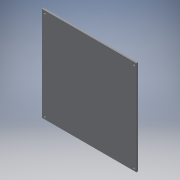
# Autodesk Inventor part: heated-bed
Saved by Autodesk Inventor 2018 (Build 220112000, 112)
## iProperties
Created: 2017-10-01
Part Number: heated-bed
Material: Generic
Document SubType Name: Modeling
Designer: Jurjen
Density: 1 g/cm^3
Appearance: Default
Author: Jurjen
Autodesk Inventor part; units mm, degrees
ref_plane "YZ Plane" through (0, 0, 0) normal (1, 0, 0) x (0, 1, 0)
ref_plane "XZ Plane" through (0, 0, 0) normal (0, 1, 0) x (-1, 0, 0)
ref_plane "XY Plane" through (0, 0, 0) normal (0, 0, 1) x (1, 0, 0)
sketch "Sketch1" plane through (0, 0, 0) normal (0, 0, 1) x (1, 0, 0)
  line L0 (-110, 110) -> (110, 110)
  line L1 (110, 110) -> (110, -110)
  line L2 (110, -110) -> (-110, -110)
  line L3 (-110, -110) -> (-110, 110)
  point P0 (0, 0)
  point P1 (110, 0)
  point P2 (0, -110)
  dimension "d0" = 220
  dimension "d1" = 220
  constraints: 8 end point, 2 midpoint, 2 parallel, 1 horizontal, 1 horizontal alignment, 1 perpendicular, 1 vertical alignment
  measures "d0" distance of L0.end L1.end
  measures "d1" distance of L1.end L2.end
extrude "Extrusion1" add sketch "Sketch1" along normal blind 4
sketch "Sketch2" plane through (0, 0, 4) normal (0, 0, 1) x (1, 0, 0)
  line L0 (110, 110) -> (-110, 110) projected
  line L1 (-110, 110) -> (-110, -110) projected
  line L2 (-110, -110) -> (110, -110) projected
  line L3 (110, -110) -> (110, 110) projected
  circle A0 centre (-104, 104) radius 1.5
  circle A1 centre (-104, -104) radius 1.5
  circle A2 centre (104, -104) radius 1.5
  circle A3 centre (104, 104) radius 1.5
  point P0 (0, 0)
  dimension "d4" = 6
  dimension "d5" = 6
  dimension "d6" = 3
  dimension "d9" = 360
  constraints: 4 centre point, 9 other
  measures "d4" distance from line of L1 A0.centre
  measures "d5" distance from line of L0 A0.centre
  measures "d6" diameter of A0
extrude "Extrusion2" cut sketch "Sketch2" against normal up to next contours A0 | A1 | A2 | A3
chamfer "Chamfer1" distance 1 angle 45 4 edges at (102.5, 104, 4) (102.5, -104, 4) (-105.5, -104, 4) (-105.5, 104, 4)
body "Solid1"
